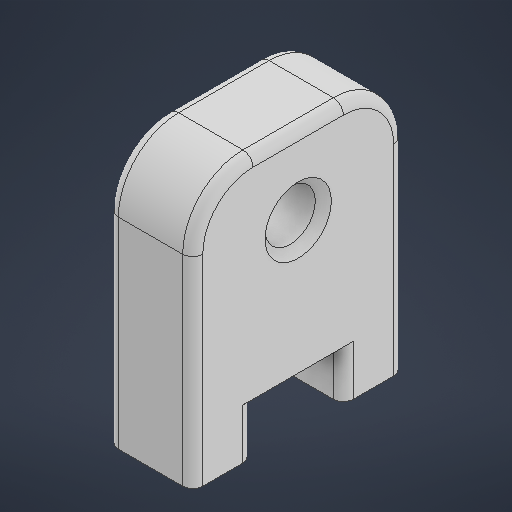
# Autodesk Inventor part: BALL SCREW MIDDLE SUPPORT
Saved by Autodesk Inventor 2025 (Build 290162000, 162)
## iProperties
Created: 2024-05-17
Part Number: BALL SCREW MIDDLE SUPPORT
Material: Generic
Document SubType Name: Modeling
Designer: zulet
Density: 1 g/cm^3
Appearance: Default
Author: zulet
Autodesk Inventor part; units mm, degrees
ref_plane "YZ Plane" through (0, 0, 0) normal (1, 0, 0) x (0, 1, 0)
ref_plane "XZ Plane" through (0, 0, 0) normal (0, 1, 0) x (-1, 0, 0)
ref_plane "XY Plane" through (0, 0, 0) normal (0, 0, 1) x (1, 0, 0)
sketch "Sketch1" plane through (0, 0, 0) normal (0, 1, 0) x (-1, 0, 0)
  line L0 (-21, -52.5) -> (21, -52.5)
  line L1 (21, -52.5) -> (21, 52.5)
  line L2 (21, 52.5) -> (-21, 52.5)
  line L3 (-21, 52.5) -> (-21, -52.5)
  line L4 (-21, -52.5) -> (21, 52.5) construction
  line L5 (21, -52.5) -> (-21, 52.5) construction
  line L6 (-11, -42.5) -> (11, -42.5) construction
  line L7 (11, -42.5) -> (11, 42.5) construction
  line L8 (11, 42.5) -> (-11, 42.5) construction
  line L9 (-11, 42.5) -> (-11, -42.5) construction
  line L10 (-11, -42.5) -> (11, 42.5) construction
  line L11 (11, -42.5) -> (-11, 42.5) construction
  line L12 (-21, -22.5) -> (21, -22.5)
  line L13 (21, -22.5) -> (21, 22.5)
  line L14 (21, 22.5) -> (-21, 22.5)
  line L15 (-21, 22.5) -> (-21, -22.5)
  line L16 (-21, -22.5) -> (21, 22.5) construction
  line L17 (21, -22.5) -> (-21, 22.5) construction
  circle A0 centre (11, 42.5) radius 3.5
  circle A1 centre (-11, 42.5) radius 3.5
  circle A2 centre (11, -42.5) radius 3.5
  circle A3 centre (-11, -42.5) radius 3.5
  point P0 (0, 0)
  dimension "d0" = 22
  dimension "d1" = 85
  dimension "d2" = 10
  dimension "d3" = 10
  dimension "d4" = 45
  dimension "d5" = 7
  dimension "d6" = 7
  dimension "d8" = 7
  dimension "d9" = 7
  constraints: 36 end point, 6 midpoint, 6 parallel, 4 centre point, 4 coincident, 3 horizontal, 3 perpendicular, 1 point on line
  measures "d0" distance of L8.end L7.end
  measures "d1" distance of L7.end L6.end
  measures "d2" distance between parallel lines of L1 L7
  measures "d3" distance between parallel lines of L6 L0
  measures "d4" distance of L12.end L13.end
  measures "d5" diameter of A0
  measures "d6" diameter of A1
  measures "d8" diameter of A2
  measures "d9" diameter of A3
extrude "Extrusion1" add sketch "Sketch1" against normal blind 25 contours L3 L12 L1 L0 | L3 L2 L1 L14
extrude "Extrusion2" add sketch "Sketch1" along normal blind 105 contours L3 L12 L1 L0 | L3 L14 L1 L12 | L3 L2 L1 L14 | A0 | A1 | A2 | A3
sketch "Sketch2" plane through (21, -25, -22.5) normal (1, 0, 0) x (0, 0, -1)
  circle A0 centre (-22.5, 91) radius 12.5
  line L0 (-45, 0) -> (-75, 0) projected
  line L1 (-22.5, 25) -> (-22.5, 91) construction
  dimension "d14" = 25
  dimension "d15" = 91
  constraints: 2 end point, 1 centre point, 1 vertical
  measures "d14" diameter of A0
  measures "d15" distance from line of L0 L1.end
extrude "Extrusion3" cut sketch "Sketch2" against normal through all
fillet "Fillet1" radius 30 2 edges at (0, 105, 52.5) (0, 105, -52.5)
fillet "Fillet2" radius 5 14 edges at (21, 96.2132, 43.7132) (21, 105, 0) (21, 96.2132, -43.7132) (21, 25, -52.5) (21, 25, 52.5) (-21, 25, 52.5) (-21, 105, 0) (-21, 96.2132, -43.7132) (-21, 25, -52.5) (-21, 96.2132, 43.7132) (21, -12.5, 22.5) (21, -12.5, -22.5) (-21, -12.5, -22.5) (-21, -12.5, 22.5)
chamfer "Chamfer1" distance 4 angle 45 2 edges at (21, 66, 12.5) (-21, 66, 12.5)
equation "\"d3\" = d2"
equation "\"d6\" = d5"
equation "\"d8\" = d5"
equation "\"d9\" = d5"
body "Solid1"
